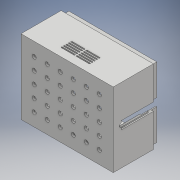
# Autodesk Inventor part: Bottom
Saved by Autodesk Inventor 2017 (Build 210142000, 142)
## iProperties
Created: 2018-02-12
Part Number: Bottom
Material: Generic
Document SubType Name: Modeling
Designer: Arjuna
Density: 1 g/cm^3
Appearance: Default
Author: Arjuna
## iProperties of the stored document Bottom_3DPrint.ipt
Created: 2018-03-05
Part Number: Bottom_3DPrint
Material: Generic
Document SubType Name: Modeling
Designer: Arjuna
Density: 1 g/cm^3
Appearance: Default
Author: Arjuna
Autodesk Inventor part; units mm, degrees
ref_plane "YZ Plane" through (0, 0, 0) normal (1, 0, 0) x (0, 1, 0)
ref_plane "XZ Plane" through (0, 0, 0) normal (0, 1, 0) x (-1, 0, 0)
ref_plane "XY Plane" through (0, 0, 0) normal (0, 0, 1) x (1, 0, 0)
sketch "Sketch1" plane through (0, 0, 0) normal (0, 1, 0) x (-1, 0, 0)
  line L0 (115, 92.5) -> (-115, 92.5)
  line L1 (-115, 92.5) -> (-115, -92.5)
  line L2 (-115, -92.5) -> (115, -92.5)
  line L3 (115, -92.5) -> (115, 92.5)
  point P0 (0, 0)
  dimension "d0" = 230
  dimension "d1" = 185
  dimension "d2" = 115
  dimension "d3" = 92.5
  constraints: 8 end point, 2 parallel, 1 horizontal, 1 perpendicular
  measures "d0" distance between parallel lines of L1 L3
  measures "d1" distance between parallel lines of L2 L0
  measures "d2" distance from line of point (0, 0) L3
  measures "d3" distance from line of point (0, 0) L0
extrude "Extrusion1" add sketch "Sketch1" along normal blind 100
sketch "Sketch3" plane through (0, 100, 0) normal (0, 1, 0) x (1, 0, 0)
  line L0 (-115, -92.5) -> (115, -92.5) projected
  line L1 (115, -92.5) -> (115, 92.5) projected
  line L2 (115, 92.5) -> (-115, 92.5) projected
  line L3 (-115, 92.5) -> (-115, -92.5) projected
  line L4 (-109.5, -87) -> (109.5, -87)
  line L5 (109.5, -87) -> (109.5, 87)
  line L6 (109.5, 87) -> (-109.5, 87)
  line L7 (-109.5, 87) -> (-109.5, -87)
  point P0 (0, 0)
  dimension "d12" = 5.5
  dimension "d13" = 5.5
  dimension "d14" = 5.5
  dimension "d15" = 5.5
  constraints: 8 end point, 2 parallel, 1 horizontal, 1 perpendicular
  measures "d12" distance between parallel lines of L4 L0
  measures "d13" distance between parallel lines of L7 L3
  measures "d14" distance between parallel lines of L2 L6
  measures "d15" distance between parallel lines of L1 L5
extrude "Extrusion3" add sketch "Sketch3" along normal blind 14 contours L7 L6 L5 L4
sketch "Sketch4" plane through (0, 114, 0) normal (0, 1, 0) x (1, 0, 0)
  line L0 (-109.5, -87) -> (109.5, -87) projected
  line L1 (109.5, -87) -> (109.5, 87) projected
  line L2 (109.5, 87) -> (-109.5, 87) projected
  line L3 (-109.5, 87) -> (-109.5, -87) projected
  line L4 (-107, -84.5) -> (107, -84.5)
  line L5 (107, -84.5) -> (107, 84.5)
  line L6 (107, 84.5) -> (-107, 84.5)
  line L7 (-107, 84.5) -> (-107, -84.5)
  point P0 (0, 0)
  dimension "d18" = 2.5
  dimension "d19" = 2.5
  dimension "d20" = 2.5
  dimension "d21" = 2.5
  constraints: 8 end point, 2 parallel, 1 horizontal, 1 perpendicular
  measures "d18" distance between parallel lines of L4 L0
  measures "d19" distance between parallel lines of L7 L3
  measures "d20" distance between parallel lines of L2 L6
  measures "d21" distance between parallel lines of L1 L5
extrude "Extrusion4" cut sketch "Sketch4" against normal blind 109 contours L7 L6 L5 L4
sketch "Sketch5" plane through (-115, 0, 92.5) normal (0, 0, 1) x (1, 0, 0)
  line L0 (0, 0) -> (230, 0) projected
  line L1 (230, 0) -> (230, 100) projected
  line L2 (0, 100) -> (230, 100) projected
  line L3 (0, 0) -> (0, 100) projected
  line L4 (115, 53) -> (115, 52)
  line L5 (115, 45.5) -> (115, 44.5)
  line L6 (115, 38) -> (115, 37)
  line L7 (115, 30.5) -> (115, 29.5)
  line L8 (115, 23) -> (115, 22)
  line L9 (118, 53) -> (118, 52)
  line L10 (118, 45.5) -> (118, 44.5)
  line L11 (118, 38) -> (118, 37)
  line L12 (118, 30.5) -> (118, 29.5)
  line L13 (118, 23) -> (118, 22)
  arc A0 (79.5, 55) -> (77.5, 53) centre (79.5, 53) ccw
  arc A1 (77.5, 22) -> (79.5, 20) centre (79.5, 22) ccw
  arc A2 (152.5, 53) -> (150.5, 55) centre (150.5, 53) ccw
  arc A3 (150.5, 20) -> (152.5, 22) centre (150.5, 22) ccw
  line L14 (79.5, 50) -> (113, 50)
  line L15 (120, 50) -> (150.5, 50)
  line L16 (150.5, 47.5) -> (120, 47.5)
  line L17 (113, 47.5) -> (79.5, 47.5)
  line L18 (79.5, 42.5) -> (113, 42.5)
  line L19 (120, 42.5) -> (150.5, 42.5)
  line L20 (150.5, 40) -> (120, 40)
  line L21 (113, 40) -> (79.5, 40)
  line L22 (79.5, 35) -> (113, 35)
  line L23 (120, 35) -> (150.5, 35)
  line L24 (150.5, 32.5) -> (120, 32.5)
  line L25 (113, 32.5) -> (79.5, 32.5)
  line L26 (79.5, 27.5) -> (113, 27.5)
  line L27 (120, 27.5) -> (150.5, 27.5)
  line L28 (150.5, 25) -> (120, 25)
  line L29 (113, 25) -> (79.5, 25)
  line L30 (79.5, 55) -> (113, 55)
  line L31 (120, 55) -> (150.5, 55)
  line L32 (79.5, 50) -> (113, 50)
  line L33 (120, 50) -> (150.5, 50)
  line L34 (79.5, 47.5) -> (113, 47.5)
  line L35 (120, 47.5) -> (150.5, 47.5)
  line L36 (79.5, 42.5) -> (113, 42.5)
  line L37 (120, 42.5) -> (150.5, 42.5)
  line L38 (79.5, 40) -> (113, 40)
  line L39 (120, 40) -> (150.5, 40)
  line L40 (79.5, 35) -> (113, 35)
  line L41 (120, 35) -> (150.5, 35)
  line L42 (79.5, 32.5) -> (113, 32.5)
  line L43 (120, 32.5) -> (150.5, 32.5)
  line L44 (79.5, 27.5) -> (113, 27.5)
  line L45 (120, 27.5) -> (150.5, 27.5)
  line L46 (79.5, 25) -> (113, 25)
  line L47 (120, 25) -> (150.5, 25)
  line L48 (77.5, 22) -> (77.5, 23)
  line L49 (77.5, 29.5) -> (77.5, 30.5)
  line L50 (77.5, 37) -> (77.5, 38)
  line L51 (77.5, 44.5) -> (77.5, 45.5)
  line L52 (77.5, 52) -> (77.5, 53)
  line L53 (118, 52) -> (118, 53)
  line L54 (115, 53) -> (115, 52)
  line L55 (118, 44.5) -> (118, 45.5)
  line L56 (115, 45.5) -> (115, 44.5)
  line L57 (115, 38) -> (115, 37)
  line L58 (118, 37) -> (118, 38)
  line L59 (118, 22) -> (118, 23)
  line L60 (118, 29.5) -> (118, 30.5)
  line L61 (115, 30.5) -> (115, 29.5)
  line L62 (115, 23) -> (115, 22)
  line L63 (152.5, 23) -> (152.5, 22)
  line L64 (152.5, 30.5) -> (152.5, 29.5)
  line L65 (152.5, 38) -> (152.5, 37)
  line L66 (152.5, 53) -> (152.5, 52)
  line L67 (152.5, 45.5) -> (152.5, 44.5)
  arc A4 (77.5, 52) -> (79.5, 50) centre (79.5, 52) ccw
  arc A5 (113, 50) -> (115, 52) centre (113, 52) ccw
  arc A6 (115, 53) -> (113, 55) centre (113, 53) ccw
  arc A7 (120, 55) -> (118, 53) centre (120, 53) ccw
  arc A8 (118, 52) -> (120, 50) centre (120, 52) ccw
  arc A9 (150.5, 50) -> (152.5, 52) centre (150.5, 52) ccw
  arc A10 (79.5, 47.5) -> (77.5, 45.5) centre (79.5, 45.5) ccw
  arc A11 (77.5, 44.5) -> (79.5, 42.5) centre (79.5, 44.5) ccw
  arc A12 (115, 45.5) -> (113, 47.5) centre (113, 45.5) ccw
  arc A13 (113, 42.5) -> (115, 44.5) centre (113, 44.5) ccw
  arc A14 (120, 47.5) -> (118, 45.5) centre (120, 45.5) ccw
  arc A15 (118, 44.5) -> (120, 42.5) centre (120, 44.5) ccw
  arc A16 (150.5, 42.5) -> (152.5, 44.5) centre (150.5, 44.5) ccw
  arc A17 (152.5, 45.5) -> (150.5, 47.5) centre (150.5, 45.5) ccw
  arc A18 (152.5, 38) -> (150.5, 40) centre (150.5, 38) ccw
  arc A19 (150.5, 35) -> (152.5, 37) centre (150.5, 37) ccw
  arc A20 (118, 37) -> (120, 35) centre (120, 37) ccw
  arc A21 (120, 40) -> (118, 38) centre (120, 38) ccw
  arc A22 (120, 32.5) -> (118, 30.5) centre (120, 30.5) ccw
  arc A23 (152.5, 30.5) -> (150.5, 32.5) centre (150.5, 30.5) ccw
  arc A24 (150.5, 27.5) -> (152.5, 29.5) centre (150.5, 29.5) ccw
  arc A25 (118, 29.5) -> (120, 27.5) centre (120, 29.5) ccw
  arc A26 (79.5, 40) -> (77.5, 38) centre (79.5, 38) ccw
  arc A27 (115, 38) -> (113, 40) centre (113, 38) ccw
  arc A28 (113, 35) -> (115, 37) centre (113, 37) ccw
  arc A29 (77.5, 37) -> (79.5, 35) centre (79.5, 37) ccw
  arc A30 (79.5, 32.5) -> (77.5, 30.5) centre (79.5, 30.5) ccw
  arc A31 (77.5, 29.5) -> (79.5, 27.5) centre (79.5, 29.5) ccw
  arc A32 (79.5, 25) -> (77.5, 23) centre (79.5, 23) ccw
  arc A33 (115, 23) -> (113, 25) centre (113, 23) ccw
  arc A34 (115, 30.5) -> (113, 32.5) centre (113, 30.5) ccw
  arc A35 (113, 27.5) -> (115, 29.5) centre (113, 29.5) ccw
  arc A36 (120, 25) -> (118, 23) centre (120, 23) ccw
  line L68 (150.5, 20) -> (120, 20)
  line L69 (113, 20) -> (79.5, 20)
  arc A37 (113, 20) -> (115, 22) centre (113, 22) ccw
  arc A38 (118, 22) -> (120, 20) centre (120, 22) ccw
  arc A39 (152.5, 23) -> (150.5, 25) centre (150.5, 23) ccw
  point P0 (115, 0)
  dimension "d52" = 34.5
  dimension "d54" = 75
  dimension "d55" = 2.5
  dimension "d56" = 7.5
  dimension "d57" = 10
  dimension "d58" = 17.5
  dimension "d59" = 22.5
  dimension "d60" = 25
  dimension "d61" = 5
  dimension "d62" = 30
  dimension "d63" = 15
  constraints: 132 end point, 116 tangent, 100 perpendicular, 80 point on circle, 55 parallel, 40 centre point, 36 equal radius, 21 collinear, 2 horizontal
  measures "d52" distance between parallel lines of L64 L60
  measures "d54" distance between parallel lines of L48 L64
  measures "d55" distance between parallel lines of L16 L33
  measures "d56" distance between parallel lines of L37 L33
  measures "d57" distance between parallel lines of L20 L33
  measures "d58" distance between parallel lines of L24 L33
  measures "d59" distance between parallel lines of L27 L33
  measures "d60" distance between parallel lines of L28 L33
  measures "d61" distance between parallel lines of L33 L31
  measures "d62" distance between parallel lines of L69 L33
  measures "d63" distance between parallel lines of L23 L33
extrude "Extrusion5" [suppressed]
sketch "Sketch6" plane through (-115, 0, 92.5) normal (0, 0, 1) x (1, 0, 0)
  line L0 (79, 21.5) -> (113.5, 21.5) construction
  line L1 (80.5, 20) -> (112, 20)
  line L2 (112, 23) -> (80.5, 23)
  arc A0 (80.5, 23) -> (80.5, 20) centre (80.5, 21.5) ccw
  arc A1 (112, 20) -> (112, 23) centre (112, 21.5) ccw
  line L3 (0, 0) -> (230, 0) projected
  line L4 (230, 0) -> (230, 100) projected
  line L5 (0, 100) -> (230, 100) projected
  line L6 (0, 0) -> (0, 100) projected
  point P0 (115, 0)
  point P1 (96.25, 21.5)
  dimension "d66" = 34.5
  dimension "d67" = 3
  dimension "d69" = 1.5
  dimension "d70" = 20
  constraints: 8 end point, 6 point on circle, 4 tangent, 2 centre point, 2 point on line, 1 horizontal, 1 midpoint, 1 parallel
  measures "d66" distance of L0.start L0.end
  measures "d67" diameter of A1
  measures "d69" horizontal distance of point (115, 0) L0.end
  measures "d70" distance between parallel lines of L3 L1
extrude "Extrusion6" cut sketch "Sketch6" against normal through all contours A0 L2 A1 L1
pattern_linear "Rectangular Pattern1" count 2 spacing 37.5 along (1, 0, 0) count 5 spacing 6 along (0, 1, 0) of "Extrusion6"
sketch "Sketch7" plane through (115, 0, 92.5) normal (1, 0, 0) x (0, 0, -1)
  line L0 (0, 0) -> (185, 0) projected
  line L1 (185, 0) -> (185, 100) projected
  line L2 (0, 100) -> (185, 100) projected
  line L3 (0, 0) -> (0, 100) projected
  circle A0 centre (92.5, 20) radius 5
  line L4 (179.5, 100) -> (5.5, 100) projected
  line L5 (179.5, 100) -> (179.5, 114) projected
  line L6 (5.5, 114) -> (179.5, 114) projected
  line L7 (5.5, 100) -> (5.5, 114) projected
  line L8 (82.5, 20) -> (102.5, 20)
  line L9 (102.5, 20) -> (102.5, 114)
  line L10 (102.5, 114) -> (82.5, 114)
  line L11 (82.5, 114) -> (82.5, 20)
  point P0 (92.5, 0)
  dimension "d79" = 10
  dimension "d82" = 20
  dimension "d83" = 10
  dimension "d84" = 20
  dimension "d93" = 185
  dimension "d94" = 92.5
  constraints: 8 end point, 2 parallel, 1 centre point, 1 horizontal, 1 perpendicular, 1 point on line
  measures "d79" diameter of A0
  measures "d82" distance of L10.end L9.end
  measures "d83" distance from line of A0.centre L11
  measures "d84" distance of point (92.5, 0) A0.centre
  measures "d93" distance of L0.start L0.end
  measures "d94" distance from line of L1 A0.centre
extrude "Extrusion7" cut sketch "Sketch7" against normal up to surface (8 mm away) contours L11 L6 L9 L2 | L2 L9 L8 A0 L11 | L8 A0 | A0 L8
sketch "Sketch8" plane through (115, 20, 10) normal (0, 0, -1) x (-1, 0, 0)
  line L0 (0, 80) -> (5.5, 80) projected
  line L1 (0, 0) -> (0, 80) projected
  line L2 (0, 0) -> (8, 0) projected
  line L3 (8, 94) -> (8, 0) projected
  line L4 (5.5, 94) -> (8, 94) projected
  line L5 (5.5, 80) -> (5.5, 94) projected
  line L6 (3, 70) -> (5.5, 70)
  line L7 (5.5, 70) -> (5.5, 55)
  line L8 (5.5, 55) -> (3, 55)
  line L9 (3, 55) -> (3, 70)
  line L10 (3, 55) -> (8, 55)
  line L11 (8, 55) -> (8, 0)
  line L12 (8, 0) -> (3, 0)
  line L13 (3, 0) -> (3, 55)
  point P0 (115, -20)
  dimension "d87" = 2.5
  dimension "d88" = 15
  dimension "d89" = 10
  dimension "d90" = 3
  dimension "d95" = 2.5
  constraints: 16 end point, 4 parallel, 2 horizontal, 2 perpendicular
  measures "d87" distance of L7.end L8.end
  measures "d88" distance between parallel lines of L8 L6
  measures "d89" distance between parallel lines of L6 L0
  measures "d90" distance between parallel lines of L9 L1
  measures "d95" distance between parallel lines of L3 L7
extrude "Extrusion8" add sketch "Sketch8" along normal blind 3 contours L13 L8 L10 L3 L2 | L9 L6 L7 L8
mirror "Mirror1" about plane through (0, 0, 0) normal (0, 0, 1) of "Extrusion8"
sketch "Sketch9" plane through (0, 5, 0) normal (0, 1, 0) x (1, 0, 0)
  line L0 (107, -84.5) -> (-107, -84.5) projected
  line L1 (107, 84.5) -> (107, -84.5) projected
  line L2 (-107, 84.5) -> (107, 84.5) projected
  line L3 (-107, -84.5) -> (-107, 84.5) projected
  circle A0 centre (-82, -59.5) radius 5
  point P0 (0, 0)
  dimension "d96" = 10
  dimension "d97" = 25
  dimension "d98" = 25
  constraints: 1 centre point
  measures "d96" diameter of A0
  measures "d97" distance from line of L3 A0.centre
  measures "d98" distance from line of L0 A0.centre
extrude "Extrusion9" cut sketch "Sketch9" against normal through all contours A0
pattern_linear "Rectangular Pattern2" count 6 spacing 32.5 along (1, 0, 0) count 5 spacing 30 along (0, 0, -1) of "Extrusion9"
equation "\"d2\" = 0.5 * d0"
equation "\"d3\" = 0.5 * d1"
equation "\"d13\" = d12"
equation "\"d14\" = d12"
equation "\"d15\" = d12"
equation "\"d19\" = d18"
equation "\"d20\" = d18"
equation "\"d21\" = d18"
equation "\"d83\" = 0.5 * d82"
equation "\"d94\" = 0.5 * d93"
equation "\"d28\" = 0.5 * d26"
equation "\"d38\" = d36"
equation "\"d39\" = d37"
equation "\"d40\" = d36"
equation "\"d41\" = d37"
equation "\"d42\" = d36"
equation "\"d43\" = d37"
equation "\"d44\" = d36"
equation "\"d47\" = 0.5 * d26"
equation "\"d26\" = 75"
equation "\"d36\" = 5"
equation "\"d37\" = 2.5"
body "Solid1"
